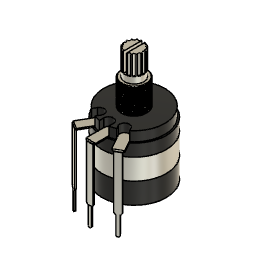
Pot_WH137-1Ak-4 (Autodesk Fusion 360 design; units mm, degrees)
Autodesk Fusion 360 part; units mm, degrees
sketch "Sketch1" plane through (0, 0, 0) normal (0, 0, 1) x (1, 0, 0)
  circle A0 centre (0, 0) radius 10
  dimension "d1" = 20
  constraint coincident A0.centre origin
  measures "d1" diameter of A0
extrude "Extrude1" add sketch "Sketch1" along normal blind 6.5 makes body 1
extrude "Extrude2" add 1 faces at (3.1852, -0.9825, 6.5) along direction (0, 0, 1) blind 6.5 separate body on bodies 1 makes body 2
extrude "Extrude3" add 1 faces at (3.1852, -0.9825, 13) along direction (0, 0, 1) blind 3.8 separate body on bodies 2 makes body 3
sketch "Sketch2" plane through (0, 0, 16.8) normal (0, 0, 1) x (-1, 0, 0)
  circle A0 centre (0, 0) radius 10
  circle A1 centre (0, 0) radius 9.5
  dimension "d8" = 19
  constraint coincident A0.centre A1.centre
  measures "d8" diameter of A1
extrude "Extrude4" add sketch "Sketch2" along normal blind 3 separate body contours A1 makes body 4
sketch "Sketch3" plane through (0, 0, 19.8) normal (0, 0, 1) x (-1, 0, 0)
  circle A0 centre (0, 0) radius 9.5
  circle A1 centre (0, 0) radius 3.875
  dimension "d11" = 7.75
  constraint coincident A0.centre A1.centre
  measures "d11" diameter of A1
extrude "Extrude5" add sketch "Sketch3" along normal blind 8 separate body contours A1 makes body 5
sketch "Sketch4" plane through (0, 0, 27.8) normal (0, 0, 1) x (-1, 0, 0)
  circle A0 centre (0, 0) radius 3.875
  circle A1 centre (0, 0) radius 2.95
  dimension "d14" = 5.9
  constraint coincident A0.centre A1.centre
  measures "d14" diameter of A1
extrude "Extrude6" add sketch "Sketch4" along normal blind 8 separate body contours A1 makes body 6
sketch "Sketch5" plane through (0, 0, 19.8) normal (0, 0, 1) x (-1, 0, 0)
  circle A0 centre (0, 0) radius 9.5
  line L0 (0, -20) -> (0, 23) construction
  line L1 (0, 0) -> (14.8868, -25.7848) construction
  line L2 (0, 0) -> (29.7737, 0) construction
  line L3 (0, 0) -> (-13.9379, 24.1411) construction
  line L4 (0, 0) -> (27.8758, 0) construction
  line L5 (0, 0) -> (-13.4629, -23.3184) construction
  line L6 (0, 0) -> (26.9258, 0) construction
  line L7 (0, 0) -> (16.9031, 29.277) construction
  line L8 (0, 0) -> (33.8061, 0) construction
  circle A1 centre (0, 0) radius 8 construction
  line L9 (0, 8) -> (-1.5, 8) construction
  line L10 (0, 8) -> (1.5, 8) construction
  arc A2 (-1.5, 8) -> (1.5, 8) centre (0, 8) ccw
  line L11 (1.5, 8) -> (1.5, 9.8864)
  line L12 (-1.5, 8) -> (-1.5, 9.8864)
  arc A3 (1.5, 9.8864) -> (-1.5, 9.8864) centre (-0.0001, 0.2512) ccw
  line L13 (-4, 6.9282) -> (-5.299, 6.1782) construction
  line L14 (-4, 6.9282) -> (-2.701, 7.6782) construction
  line L15 (-2.701, 7.6782) -> (-3.6441, 9.3118)
  line L16 (-5.299, 6.1782) -> (-6.2422, 7.8118)
  line L17 (-5.299, 6.1782) -> (-3.4126, 6.1782) construction
  arc A4 (-5.299, 6.1782) -> (-2.701, 7.6782) centre (-4.185, 7.2487) ccw
  arc A5 (-3.6441, 9.3118) -> (-6.2422, 7.8118) centre (-0.1254, 0.2176) ccw
  line L18 (4, 6.9282) -> (5.299, 6.1782) construction
  line L19 (4, 6.9282) -> (2.701, 7.6782) construction
  line L20 (5.299, 6.1782) -> (6.2421, 7.8117)
  line L21 (5.299, 6.1782) -> (7.1852, 6.1782) construction
  line L22 (2.701, 7.6782) -> (3.6441, 9.3117)
  line L23 (2.701, 7.6782) -> (4.5872, 7.6782) construction
  arc A6 (6.2421, 7.8117) -> (3.6441, 9.3117) centre (0.1255, 0.2175) ccw
  arc A7 (2.701, 7.6782) -> (5.299, 6.1782) centre (4, 6.9282) ccw
  dimension "d17" = 60
  dimension "d18" = 120
  dimension "d19" = 120
  dimension "d20" = 60
  dimension "d21" = 16
  dimension "d22" = 1.5
  dimension "d23" = 1.5
  dimension "d32" = 1.5
  dimension "d33" = 1.5
  dimension "d34" = 120
  dimension "d37" = 1.5
  dimension "d38" = 1.5
  dimension "d39" = 60
  dimension "d40" = 60
  constraint vertical L0
  constraint horizontal L2
  constraint coincident A0.centre L1.start
  constraint horizontal L4
  constraint horizontal L6
  constraint horizontal L8
  constraint coincident L0 L9.start
  constraint coincident A1 L9.start
  constraint perpendicular L0 L9
  constraint perpendicular L0 L10
  constraint tangent A2 L11
  constraint tangent A2 L12
  constraint tangent A0 A3
  constraint coincident L3 L13.start
  constraint coincident A1 L13.start
  constraint perpendicular L3 L13
  constraint perpendicular L3 L14
  constraint perpendicular L14 L15
  constraint horizontal L17
  constraint tangent A0 A5
  constraint coincident A1 L18.start
  constraint coincident L7 L18.start
  constraint perpendicular L7 L18
  constraint perpendicular L7 L19
  constraint horizontal L21
  constraint horizontal L23
  constraint tangent A0 A6
  constraint tangent L22 A7
  measures "d17" angle of L1 L2
  measures "d18" angle of L3 L4
  measures "d19" angle of L5 L6
  measures "d20" angle of L7 L8
  measures "d21" diameter of A1
  measures "d22" distance of L9.start L9.end
  measures "d23" distance of L9.start L10.end
  measures "d32" distance of L13.start L13.end
  measures "d33" distance of L13.start L14.end
  measures "d34" angle of L16 L17
  measures "d37" distance of L18.start L18.end
  measures "d38" distance of L18.start L19.end
  measures "d39" angle of L20 L21
  measures "d40" angle of L22 L23
extrude "Extrude7" cut sketch "Sketch5" against normal blind 3 contours A0 A2 L11 L12 | A0 L11 L12 A3 bodies 4
sketch "Sketch8" plane through (0, 0, 35.8) normal (0, 0, 1) x (-1, 0, 0)
  circle A0 centre (0, 0) radius 2.95
  line L0 (-0.5, 2.9073) -> (-0.5, -2.9073)
  line L1 (0.5, -2.9073) -> (0.5, 2.9073)
  line L2 (0.5, 2.9073) -> (-0.5, -2.9073) construction
  line L3 (-0.5, 2.9073) -> (0.5, -2.9073) construction
  dimension "d29" = 1
  constraint parallel L0 L1
  constraint coincident L2 A0.centre
  constraint coincident L3 A0.centre
  constraint coincident A0.centre origin
  constraint coincident A0 L0.start
  measures "d29" distance of L0.end L1.start
extrude "Extrude9" cut sketch "Sketch8" against normal blind 6 contours A0 L0 L1 bodies 6
extrude "Extrude10" cut sketch "Sketch5" against normal blind 3 contours A0 L15 L16 A5 | A0 L15 L16 A4 bodies 4
extrude "Extrude11" cut sketch "Sketch5" against normal blind 3 contours A0 L20 L22 A7 | A0 L20 L22 A6 bodies 4
sketch "Sketch11" plane through (0, 0, 35.8) normal (0, 0, 1) x (-1, 0, 0)
  line L0 (-0.5, -2.9073) -> (-0.5, 2.9073)
  arc A0 (-0.5, 2.9073) -> (-0.5, -2.9073) centre (0, 0) ccw
  arc A1 (-1.4839, 2.5496) -> (-0.7461, 2.8541) centre (-1.1253, 2.7269) ccw
  dimension "d47" = 0.8
  constraint coincident A0 A1.centre
  constraint coincident A0 A1.end
  constraint coincident A0 A1.start
  measures "d47" diameter of A1
extrude "Extrude12" cut sketch "Sketch11" against normal blind 6 contours A0 A1 bodies 6
pattern_circular "C-Pattern1" count 16 over 360 about axis through (0, 0, 35.8) along (0, 0, 1) of "Extrude12"
fillet "Fillet2" radius 0.2 1 edges at (3.6128, 1.4013, 27.8) on bodies 5
thread "Thread1" "ISO Metric profile 8.0 M8x0.5 6g" major diameter 7.927 minor diameter 7.3505 pitch 0.5 angle 60 modelled right hand crest width 0.0685 on face at (-3.8557, 0.3858, 25) crest through (-3.9635, 0, 19.675) on bodies 5
sketch "Sketch12" plane through (0, 0, 16.8) normal (0, 0, 1) x (-1, 0, 0)
  circle A0 centre (0, 0) radius 10
  line L0 (1.5, 8) -> (1.5, 9.8864)
  arc A1 (-1.5, 8) -> (1.5, 8) centre (0, 8) ccw
  line L1 (-1.5, 8) -> (-1.5, 9.8864)
  arc A2 (1.5, 9.8864) -> (1.3761, 9.9049) centre (-0.0001, 0.2512) ccw
  arc A3 (-1.3801, 9.9043) -> (-1.5, 9.8864) centre (-0.0001, 0.2512) ccw
  line L2 (1.5, 9.8864) -> (1.5, 13.8864)
  line L3 (-1.5, 9.8864) -> (-1.5, 13.8864)
  line L4 (1.5, 13.8864) -> (-1.5, 13.8864)
  line L5 (5.299, 6.1782) -> (6.2421, 7.8117)
  line L6 (2.701, 7.6782) -> (3.6441, 9.3117)
  arc A4 (2.701, 7.6782) -> (5.299, 6.1782) centre (4, 6.9282) ccw
  arc A5 (-5.299, 6.1782) -> (-2.701, 7.6782) centre (-4.185, 7.2487) ccw
  line L7 (-2.701, 7.6782) -> (-3.6441, 9.3118)
  line L8 (-5.299, 6.1782) -> (-6.2422, 7.8118)
  line L9 (6.2421, 7.8117) -> (8.2421, 11.2758)
  line L10 (3.6441, 9.3117) -> (5.6441, 12.7758)
  line L11 (8.2421, 11.2758) -> (5.6441, 12.7758)
  line L12 (-3.6441, 9.3118) -> (-5.6441, 12.7759)
  line L13 (-6.2422, 7.8118) -> (-8.2422, 11.2759)
  line L14 (-8.2422, 11.2759) -> (-5.6441, 12.7759)
  dimension "d56" = 4
  dimension "d57" = 4
  dimension "d60" = 4
  dimension "d61" = 4
  dimension "d62" = 4
  dimension "d64" = 4
  constraint tangent L0 A1
  constraint tangent A1 L1
  constraint coincident A0 A2.end
  constraint coincident A0 A3.start
  constraint concentric A2 A3
  constraint parallel L0 L2
  constraint parallel L1 L3
  constraint tangent L6 A4
  constraint parallel L5 L9
  constraint parallel L6 L10
  constraint parallel L7 L12
  constraint parallel L8 L13
  measures "d56" distance of L0.end L2.end
  measures "d57" distance of L1.end L3.end
  measures "d60" distance of L5.end L9.end
  measures "d61" distance of L6.end L10.end
  measures "d62" distance of L7.end L12.end
  measures "d64" distance of L8.end L13.end
extrude "Extrude14" add sketch "Sketch12" along normal blind 0.4 separate body contours A0 L0 A1 L1 A2 A3 | A0 L2 L3 L4 | A0 L9 L10 L11 | A0 L5 L6 A4 L9 L10 | A0 A5 L7 L8 L12 L13 | A0 L12 L13 L14 makes body 7 at (-0.4587, -12.5592, 16.8) makes body 8 at (-5.5291, -10.5766, 16.8) makes body 9 at (5.5291, -10.5767, 16.8)
sketch "Sketch13" plane through (0, 0, 16.8) normal (0, 0, 1) x (-1, 0, 0)
  line L0 (-1.0001, 13.8864) -> (0.9999, 13.8864)
  line L1 (0.9999, 13.8864) -> (0.9999, 13.4864)
  line L2 (0.9999, 13.4864) -> (-1.0001, 13.4864)
  line L3 (-1.0001, 13.4864) -> (-1.0001, 13.8864)
  line L4 (6.0833, 12.522) -> (7.8188, 11.5281)
  line L5 (7.8188, 11.5281) -> (7.62, 11.181)
  line L6 (7.62, 11.181) -> (5.8845, 12.1749)
  line L7 (5.8845, 12.1749) -> (6.0833, 12.522)
  line L8 (-7.0849, 12.2502) -> (-6.0849, 12.2502) construction
  line L9 (-7.8183, 11.5204) -> (-6.0785, 12.5068)
  line L10 (-6.0785, 12.5068) -> (-5.8812, 12.1588)
  line L11 (-7.8183, 11.5204) -> (-7.6211, 11.1724)
  line L12 (-7.6211, 11.1724) -> (-5.8812, 12.1588)
  dimension "d65" = 2
  dimension "d66" = 0.4
  dimension "d69" = 2
  dimension "d70" = 0.4
  dimension "d71" = 2
  dimension "d76" = 2
  dimension "d77" = 0.4
  dimension "d78" = 0.4
  dimension "d79" = 2
  constraint horizontal L0
  constraint vertical L1
  constraint horizontal L2
  constraint vertical L3
  constraint perpendicular L4 L5
  constraint perpendicular L5 L6
  constraint horizontal L8
  constraint perpendicular L9 L10
  constraint perpendicular L9 L11
  constraint perpendicular L11 L12
  measures "d65" distance of L0.start L0.end
  measures "d66" distance of L0.start L2.end
  measures "d69" distance of L4.start L4.end
  measures "d70" distance of L4.end L5.end
  measures "d71" distance of L5.end L6.end
  measures "d76" distance of L9.start L9.end
  measures "d77" distance of L9.end L10.end
  measures "d78" distance of L9.start L11.end
  measures "d79" distance of L11.end L10.end
extrude "Extrude15" add sketch "Sketch13" against normal blind 17 bodies 7 8 9
chamfer "Chamfer1" distance 0.4 angle 45 6 edges at (-5.6441, -12.7758, 17) (-8.2421, -11.2758, 17) (1.5, -13.8864, 17) (-1.5, -13.8864, 17) (8.2422, -11.2759, 17) (5.6441, -12.7759, 17) on bodies 7 8 9
fillet "Fillet4" radius 0.3 3 edges at (0, -13.8864, 17.2) (-6.9431, -12.0258, 17.2) (6.9432, -12.0259, 17.2) on bodies 7 8 9
sketch "Sketch14" plane through (0, 0, -0.2) normal (0, 0, -1) x (1, 0, 0)
  line L0 (-7.62, 11.181) -> (-5.8845, 12.1749)
  line L1 (-5.8845, 12.1749) -> (-6.0833, 12.522)
  line L2 (-6.0833, 12.522) -> (-7.8188, 11.5281)
  line L3 (-7.8188, 11.5281) -> (-7.62, 11.181)
  line L4 (-7.62, 11.181) -> (-6.0833, 12.522) construction
  line L5 (-7.8188, 11.5281) -> (-5.8845, 12.1749) construction
  line L6 (-1, 13.5) -> (0.9979, 13.8817) construction
  line L7 (-1, 13.88) -> (1, 13.5) construction
  line L8 (6.0818, 12.5081) -> (7.6195, 11.1745) construction
  line L9 (7.8176, 11.5197) -> (5.88, 12.16) construction
  line L10 (6.5135, 12.2602) -> (6.3162, 11.9122)
  line L11 (6.0785, 12.5068) -> (5.8812, 12.1588)
  line L12 (6.5135, 12.2602) -> (7.3834, 11.767)
  line L13 (6.3162, 11.9122) -> (7.1861, 11.419)
  line L14 (7.1861, 11.419) -> (7.3834, 11.767)
  line L15 (-0.5, 13.88) -> (0.5, 13.88)
  line L16 (0.5, 13.88) -> (0.5, 13.48)
  line L17 (0.5, 13.48) -> (-0.5, 13.48)
  line L18 (-0.5, 13.48) -> (-0.5, 13.88)
  line L19 (-7.3849, 11.7766) -> (-7.1861, 11.4295)
  line L20 (-7.8188, 11.5281) -> (-7.62, 11.181)
  line L21 (-7.3849, 11.7766) -> (-6.5171, 12.2735)
  line L22 (-7.1861, 11.4295) -> (-6.3184, 11.9264)
  line L23 (-6.3184, 11.9264) -> (-6.5171, 12.2735)
  dimension "d87" = 0.4
  dimension "d88" = 1
  dimension "d89" = 1
  dimension "d92" = 1
  dimension "d93" = 0.4
  dimension "d94" = 0.4
  dimension "d95" = 1
  dimension "d96" = 1
  constraint coincident L0.start L3.end
  constraint coincident L1.end L2.start
  constraint coincident L2.end L3.start
  constraint coincident L0.end L1.start
  constraint parallel L10 L11
  constraint perpendicular L10 L12
  constraint perpendicular L10 L13
  constraint horizontal L15
  constraint vertical L16
  constraint horizontal L17
  constraint vertical L18
  constraint parallel L19 L20
  constraint perpendicular L19 L21
  constraint perpendicular L19 L22
  measures "d87" distance of L10.start L10.end
  measures "d88" distance of L10.start L12.end
  measures "d89" distance of L10.end L13.end
  measures "d92" distance of L15.start L15.end
  measures "d93" distance of L15.start L17.end
  measures "d94" distance of L19.start L19.end
  measures "d95" distance of L19.start L21.end
  measures "d96" distance of L19.end L22.end
extrude "Extrude16" add sketch "Sketch14" along normal blind 6 contours L0 L2 L19 L21 L22 L23 | L10 L12 L13 L14 | L15 L16 L17 L18 bodies 7 8 9
fillet "Fillet5" radius 0.6 6 edges at (1.0001, -13.6864, -0.2) (-0.9999, -13.6864, -0.2) (-5.9839, -12.3485, -0.2) (-7.7194, -11.3545, -0.2) (7.7197, -11.3464, -0.2) (5.9799, -12.3328, -0.2) on bodies 7 8 9
fillet "Fillet6" radius 0.5 6 edges at (-0.5, -13.68, -6.2) (0.5, -13.68, -6.2) (-7.2855, -11.603, -6.2) (-6.4177, -12.1, -6.2) (6.4148, -12.0862, -6.2) (7.2847, -11.593, -6.2) on bodies 7 8 9
sketch "Sketch15" plane through (0, 0, 0) normal (0, 0, -1) x (1, 0, 0)
  circle A0 centre (0, 0) radius 10
  line L0 (14, 0) -> (-13, 0) construction
  line L1 (0, 0) -> (21.2292, 0) construction
  circle A1 centre (0, 0) radius 4 construction
  line L2 (0, 0) -> (3.8637, -1.0353) construction
  line L3 (0, 0) -> (-3.8637, -1.0353) construction
  line L4 (-3.9272, 0.4767) -> (-3.4063, -2.4778)
  line L5 (-3.9272, 0.4767) -> (-11, 0.4767) construction
  line L6 (-3.4063, -2.4778) -> (-3.8002, -2.5472)
  line L7 (-3.8002, -2.5472) -> (-4.3211, 0.4072)
  line L8 (-4.3211, 0.4072) -> (-3.9272, 0.4767)
  line L9 (-3.8002, -2.5472) -> (-3.9272, 0.4767) construction
  line L10 (-4.3211, 0.4072) -> (-3.4063, -2.4778) construction
  line L11 (-3.8637, -1.0353) -> (-3.6667, -1.0005) construction
  line L12 (4.3211, 0.4072) -> (3.8002, -2.5472)
  line L13 (4.3211, 0.4072) -> (17.2483, 0.4072) construction
  line L14 (3.8002, -2.5472) -> (3.4063, -2.4778)
  line L15 (3.4063, -2.4778) -> (3.9272, 0.4767)
  line L16 (3.9272, 0.4767) -> (4.3211, 0.4072)
  line L17 (4.3211, 0.4072) -> (3.4063, -2.4778) construction
  line L18 (3.8002, -2.5472) -> (3.9272, 0.4767) construction
  line L19 (3.8637, -1.0353) -> (3.6667, -1.0005) construction
  dimension "d106" = 8
  dimension "d115" = 80
  dimension "d116" = 3
  dimension "d117" = 0.4
  dimension "d118" = 3
  dimension "d129" = 100
  dimension "d130" = 3
  dimension "d131" = 0.4
  dimension "d132" = 3
  constraint horizontal L0
  constraint horizontal L1
  constraint coincident A0.centre L1.start
  constraint coincident A1 L2.end
  constraint coincident A1 L3.end
  constraint horizontal L5
  constraint perpendicular L4 L6
  constraint perpendicular L6 L7
  constraint midpoint L9 L3.end
  constraint midpoint L4 L11.end
  constraint horizontal L13
  constraint perpendicular L12 L14
  constraint perpendicular L14 L15
  constraint midpoint L18 L2.end
  constraint midpoint L15 L19.end
  measures "d106" diameter of A1
  measures "d115" angle of L4 L5
  measures "d116" distance of L4.start L4.end
  measures "d117" distance of L4.end L6.end
  measures "d118" distance of L6.end L7.end
  measures "d129" angle of L12 L13
  measures "d130" distance of L12.start L12.end
  measures "d131" distance of L12.end L14.end
  measures "d132" distance of L14.end L15.end
extrude "Extrude17" add sketch "Sketch15" along normal blind 4 separate body contours L4 L6 L7 L8 | L12 L14 L15 L16 makes body 10 at (-4.1475, 0.5776, -2.6667) makes body 11 at (4.1475, 0.5776, -1.3333)
fillet "Fillet7" radius 1.5 4 edges at (-3.6032, 2.5125, -4) (-4.1242, -0.4419, -4) (3.6032, 2.5125, -4) (4.1242, -0.4419, -4) on bodies 10 11
sketch "Sketch16" plane through (-3.7273, 0.6572, 0) normal (0.984808, -0.173648, 0) x (0.173648, 0.984808, 0)
  arc A0 (-1.1514, -2.5) -> (1.8486, -2.5) centre (0.3486, -2.5) ccw
  line L0 (1.8486, -2.5) -> (1.8486, 0)
  line L1 (1.8486, 0) -> (-1.1514, 0)
  line L2 (-1.1514, 0) -> (-1.1514, -2.5)
  circle A1 centre (0.3486, -2.5) radius 1
  dimension "d123" = 2
  constraint concentric A0 A1
  measures "d123" diameter of A1
extrude "Extrude18" cut sketch "Sketch16" against normal blind 0.4 contours A1 bodies 10
sketch "Sketch19" plane through (3.7273, 0.6572, 0) normal (-0.984808, -0.173648, 0) x (0.173648, -0.984808, 0)
  arc A0 (-1.8486, -2.5) -> (1.1514, -2.5) centre (-0.3486, -2.5) ccw
  line L0 (1.1514, -2.5) -> (1.1514, 0)
  line L1 (1.1514, 0) -> (-1.8486, 0)
  line L2 (-1.8486, 0) -> (-1.8486, -2.5)
  circle A1 centre (-0.3486, -2.5) radius 1
  dimension "d133" = 2
  constraint concentric A0 A1
  measures "d133" diameter of A1
extrude "Extrude20" cut sketch "Sketch19" against normal blind 1.4 contours A1 bodies 11
